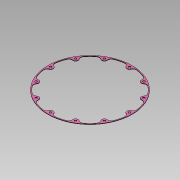
# Autodesk Inventor part: capsule.gasket
Saved by Autodesk Inventor 2011 (Build 150239000, 239)
## iProperties
Created: 2011-01-27
Part Number: capsule.gasket
Document SubType Name: Modeling
Designer: Casey
Density: 1 g/cm^3
Author: Casey
Autodesk Inventor part; units mm, degrees
ref_plane "YZ Plane" through (0, 0, 0) normal (1, 0, 0) x (0, 1, 0)
ref_plane "XZ Plane" through (0, 0, 0) normal (0, 1, 0) x (-1, 0, 0)
ref_plane "XY Plane" through (0, 0, 0) normal (0, 0, 1) x (1, 0, 0)
sketch "Sketch1" plane through (0, 0, 0) normal (0, 0, 1) x (1, 0, 0)
  circle A0 centre (39.8372, -23) radius 1.2295
  circle A1 centre (23, -39.8372) radius 1.2295
  circle A2 centre (0, -46) radius 1.2295
  circle A3 centre (-23, -39.8372) radius 1.2295
  circle A4 centre (-39.8372, -23) radius 1.2295
  circle A5 centre (-46, 0) radius 1.2295
  circle A6 centre (-39.8372, 23) radius 1.2295
  circle A7 centre (-23, 39.8372) radius 1.2295
  circle A8 centre (0, 46) radius 1.2295
  circle A9 centre (23, 39.8372) radius 1.2295
  circle A10 centre (39.8372, 23) radius 1.2295
  circle A11 centre (46, 0) radius 1.2295
  arc A12 (29.9143, -37.5385) -> (37.5385, -29.9143) centre (0, 0) ccw
  arc A13 (24.8949, -37.5114) -> (29.9143, -37.5385) centre (27.4214, -34.4103) ccw
  arc A14 (24.8949, -37.5114) -> (20.0383, -40.3153) centre (23, -39.8372) ccw
  arc A15 (17.5521, -44.6757) -> (20.0383, -40.3153) centre (16.0895, -40.9528) ccw
  arc A16 (7.1373, -47.4664) -> (17.5521, -44.6757) centre (0, 0) ccw
  arc A17 (2.8039, -44.9332) -> (7.1373, -47.4664) centre (6.5425, -43.5109) ccw
  arc A18 (2.8039, -44.9332) -> (-2.8039, -44.9332) centre (0, -46) ccw
  arc A19 (-7.1373, -47.4664) -> (-2.8039, -44.9332) centre (-6.5425, -43.5109) ccw
  arc A20 (-17.5521, -44.6757) -> (-7.1373, -47.4664) centre (0, 0) ccw
  arc A21 (-20.0383, -40.3153) -> (-17.5521, -44.6757) centre (-16.0895, -40.9528) ccw
  arc A22 (-20.0383, -40.3153) -> (-24.8949, -37.5114) centre (-23, -39.8372) ccw
  arc A23 (-29.9143, -37.5385) -> (-24.8949, -37.5114) centre (-27.4214, -34.4103) ccw
  arc A24 (-37.5385, -29.9143) -> (-29.9143, -37.5385) centre (0, 0) ccw
  arc A25 (-37.5114, -24.8949) -> (-37.5385, -29.9143) centre (-34.4103, -27.4214) ccw
  arc A26 (-37.5114, -24.8949) -> (-40.3153, -20.0383) centre (-39.8372, -23) ccw
  arc A27 (-44.6757, -17.5521) -> (-40.3153, -20.0383) centre (-40.9528, -16.0895) ccw
  arc A28 (-47.4664, -7.1373) -> (-44.6757, -17.5521) centre (0, 0) ccw
  arc A29 (-44.9332, -2.8039) -> (-47.4664, -7.1373) centre (-43.5109, -6.5425) ccw
  arc A30 (-44.9332, -2.8039) -> (-44.9332, 2.8039) centre (-46, 0) ccw
  arc A31 (-47.4664, 7.1373) -> (-44.9332, 2.8039) centre (-43.5109, 6.5425) ccw
  arc A32 (-44.6757, 17.5521) -> (-47.4664, 7.1373) centre (0, 0) ccw
  arc A33 (-40.3153, 20.0383) -> (-44.6757, 17.5521) centre (-40.9528, 16.0895) ccw
  arc A34 (-40.3153, 20.0383) -> (-37.5114, 24.8949) centre (-39.8372, 23) ccw
  arc A35 (-37.5385, 29.9143) -> (-37.5114, 24.8949) centre (-34.4103, 27.4214) ccw
  arc A36 (-29.9143, 37.5385) -> (-37.5385, 29.9143) centre (0, 0) ccw
  arc A37 (-24.8949, 37.5114) -> (-29.9143, 37.5385) centre (-27.4214, 34.4103) ccw
  arc A38 (-24.8949, 37.5114) -> (-20.0383, 40.3153) centre (-23, 39.8372) ccw
  arc A39 (-17.5521, 44.6757) -> (-20.0383, 40.3153) centre (-16.0895, 40.9528) ccw
  arc A40 (-7.1373, 47.4664) -> (-17.5521, 44.6757) centre (0, 0) ccw
  arc A41 (-2.8039, 44.9332) -> (-7.1373, 47.4664) centre (-6.5425, 43.5109) ccw
  arc A42 (-2.8039, 44.9332) -> (2.8039, 44.9332) centre (0, 46) ccw
  arc A43 (7.1373, 47.4664) -> (2.8039, 44.9332) centre (6.5425, 43.5109) ccw
  arc A44 (17.5521, 44.6757) -> (7.1373, 47.4664) centre (0, 0) ccw
  arc A45 (20.0383, 40.3153) -> (17.5521, 44.6757) centre (16.0895, 40.9528) ccw
  arc A46 (20.0383, 40.3153) -> (24.8949, 37.5114) centre (23, 39.8372) ccw
  arc A47 (29.9143, 37.5385) -> (24.8949, 37.5114) centre (27.4214, 34.4103) ccw
  arc A48 (37.5385, 29.9143) -> (29.9143, 37.5385) centre (0, 0) ccw
  arc A49 (37.5114, 24.8949) -> (37.5385, 29.9143) centre (34.4103, 27.4214) ccw
  arc A50 (37.5114, 24.8949) -> (40.3153, 20.0383) centre (39.8372, 23) ccw
  arc A51 (44.6757, 17.5521) -> (40.3153, 20.0383) centre (40.9528, 16.0895) ccw
  arc A52 (47.4664, 7.1373) -> (44.6757, 17.5521) centre (0, 0) ccw
  arc A53 (44.9332, 2.8039) -> (47.4664, 7.1373) centre (43.5109, 6.5425) ccw
  arc A54 (44.9332, 2.8039) -> (44.9332, -2.8039) centre (46, 0) ccw
  arc A55 (47.4664, -7.1373) -> (44.9332, -2.8039) centre (43.5109, -6.5425) ccw
  arc A56 (44.6757, -17.5521) -> (47.4664, -7.1373) centre (0, 0) ccw
  arc A57 (40.3153, -20.0383) -> (44.6757, -17.5521) centre (40.9528, -16.0895) ccw
  arc A58 (40.3153, -20.0383) -> (37.5114, -24.8949) centre (39.8372, -23) ccw
  arc A59 (37.5385, -29.9143) -> (37.5114, -24.8949) centre (34.4103, -27.4214) ccw
  circle A60 centre (0, 0) radius 49
  constraints: 96 point on circle, 61 centre point
extrude "Extrusion1" add sketch "Sketch1" along normal blind 0.5
body "Solid1"
